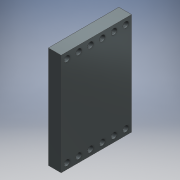
# Autodesk Inventor part: batteryholder
Saved by Autodesk Inventor 2016 (Build 200138000, 138)
## iProperties
Created: 2017-01-15
Part Number: batteryholder
Material: Generic
Document SubType Name: Modeling
Designer: hesaon
Density: 1 g/cm^3
Appearance: Default
Author: hesaon
Autodesk Inventor part; units mm, degrees
ref_plane "YZ Plane" through (0, 0, 0) normal (1, 0, 0) x (0, 1, 0)
ref_plane "XZ Plane" through (0, 0, 0) normal (0, 1, 0) x (-1, 0, 0)
ref_plane "XY Plane" through (0, 0, 0) normal (0, 0, 1) x (1, 0, 0)
sketch "Sketch1" plane through (0, 0, 0) normal (0, 1, 0) x (-1, 0, 0)
  line L0 (0, 0) -> (0, -104)
  line L1 (0, 0) -> (13, 0)
  line L2 (13, 0) -> (13, -12)
  line L3 (13, -12) -> (5, -12)
  line L4 (5, -12) -> (5, -92)
  line L5 (5, -92) -> (13, -92)
  line L6 (13, -92) -> (13, -104)
  line L7 (13, -104) -> (0, -104)
  dimension "d0" = 104
  dimension "d1" = 13
  dimension "d2" = 12
  dimension "d3" = 8
  dimension "d4" = 80
  dimension "d5" = 8
  constraints: 16 end point, 3 perpendicular, 2 point on line, 1 horizontal, 1 parallel, 1 vertical
  measures "d0" distance of L0.start L0.end
  measures "d1" distance of L0.start L1.end
  measures "d2" distance of L1.end L2.end
  measures "d3" distance of L2.end L3.end
  measures "d4" distance of L3.end L4.end
  measures "d5" distance of L4.end L5.end
extrude "Extrusion1" add sketch "Sketch1" along normal blind 72
sketch "Sketch3" plane through (-5, 0, -92) normal (-1, 0, 0) x (0, 0, 1)
  line L0 (0, 0) -> (80, 0) projected
  line L1 (0, 0) -> (80, 0) projected
  line L2 (80, 0) -> (80, 72) projected
  line L3 (0, 72) -> (80, 72) projected
  line L4 (0, 0) -> (0, 72) projected
  line L5 (0, 0) -> (0, 72) projected
  line L6 (80, 0) -> (0, 0)
  line L7 (0, 0) -> (0, 8)
  line L8 (0, 8) -> (80, 8)
  line L9 (80, 8) -> (80, 0)
  line L10 (80, 0) -> (80, 72) projected
  line L11 (80, 72) -> (0, 72)
  line L12 (0, 72) -> (0, 64)
  line L13 (0, 64) -> (80, 64)
  line L14 (80, 64) -> (80, 72)
  point P0 (92, 0)
  dimension "d14" = 8
  dimension "d15" = 8
  constraints: 16 end point, 4 parallel, 2 horizontal, 2 perpendicular, 2 point on line
  measures "d14" distance of L6.end L7.end
  measures "d15" distance of L12.end L11.end
extrude "Extrusion3" add sketch "Sketch3" along normal blind 8 contours L4 L8 L2 L0 | L4 L3 L2 L13
sketch "Sketch4" plane through (-13, 0, -104) normal (-1, 0, 0) x (0, 0, 1)
  circle A0 centre (98, 66) radius 3
  line L0 (0, 72) -> (104, 72) projected
  line L1 (0, 0) -> (0, 72) projected
  line L2 (0, 0) -> (104, 0) projected
  line L3 (104, 0) -> (104, 72) projected
  line L4 (12, 64) -> (92, 64) projected
  line L5 (92, 8) -> (92, 64) projected
  line L6 (92, 8) -> (12, 8) projected
  line L7 (12, 8) -> (12, 64) projected
  circle A1 centre (98, 54) radius 3
  circle A2 centre (98, 42) radius 3
  circle A3 centre (98, 30) radius 3
  circle A4 centre (98, 18) radius 3
  circle A5 centre (6, 6) radius 3
  circle A6 centre (98, 6) radius 3
  circle A7 centre (6, 66) radius 3
  circle A8 centre (6, 54) radius 3
  circle A9 centre (6, 42) radius 3
  circle A10 centre (6, 30) radius 3
  circle A11 centre (6, 18) radius 3
  point P0 (104, 0)
  dimension "d18" = 6
  dimension "d19" = 6
  dimension "d20" = 6
  dimension "d21" = 6
  dimension "d22" = 6
  dimension "d23" = 6
  dimension "d24" = 6
  dimension "d25" = 6
  dimension "d26" = 12
  dimension "d27" = 12
  dimension "d28" = 12
  dimension "d29" = 12
  dimension "d30" = 12
  dimension "d31" = 6
  dimension "d32" = 6
  dimension "d33" = 6
  dimension "d34" = 6
  dimension "d35" = 6
  dimension "d36" = 6
  dimension "d37" = 6
  dimension "d38" = 6
  dimension "d39" = 12
  dimension "d40" = 12
  dimension "d41" = 12
  dimension "d42" = 12
  dimension "d43" = 12
  constraints: 12 centre point, 10 vertical alignment
  measures "d18" diameter of A0
  measures "d19" distance from line of L0 A0.centre
  measures "d20" distance from line of L5 A0.centre
  measures "d21" diameter of A1
  measures "d22" diameter of A2
  measures "d23" diameter of A3
  measures "d24" diameter of A4
  measures "d25" diameter of A5
  measures "d26" distance of A1.centre A0.centre
  measures "d27" distance of A2.centre A1.centre
  measures "d28" distance of A3.centre A2.centre
  measures "d29" distance of A4.centre A3.centre
  measures "d30" distance of A6.centre A4.centre
  measures "d31" diameter of A6
  measures "d32" diameter of A7
  measures "d33" diameter of A8
  measures "d34" diameter of A9
  measures "d35" diameter of A10
  measures "d36" diameter of A11
  measures "d37" distance from line of L1 A7.centre
  measures "d38" distance from line of L0 A7.centre
  measures "d39" distance of A7.centre A8.centre
  measures "d40" distance of A8.centre A9.centre
  measures "d41" distance of A10.centre A9.centre
  measures "d42" distance of A10.centre A11.centre
  measures "d43" distance of A5.centre A11.centre
extrude "Extrusion4" cut sketch "Sketch4" against normal up to next contours A0 | A1 | A2 | A3 | A4 | A5 | A6 | A7 | A8 | A9 | A10 | A11
body "Solid1"
